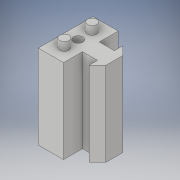
# Autodesk Inventor part: Grab Rail v2
Saved by Autodesk Inventor 2018 (Build 220112000, 112)
## iProperties
Created: 2019-12-11
Part Number: Grab Rail v2
Material: Generic
Document SubType Name: Modeling
Designer: AOFUser
Density: 1 g/cm^3
Appearance: Default
Author: AOFUser
Autodesk Inventor part; units mm, degrees
ref_plane "YZ Plane" through (0, 0, 0) normal (1, 0, 0) x (0, 1, 0)
ref_plane "XZ Plane" through (0, 0, 0) normal (0, 1, 0) x (-1, 0, 0)
ref_plane "XY Plane" through (0, 0, 0) normal (0, 0, 1) x (1, 0, 0)
sketch "Sketch1" plane through (0, 0, 0) normal (0, 1, 0) x (-1, 0, 0)
  line L0 (0, 0) -> (7.62, 0)
  line L1 (7.62, 0) -> (7.62, -16.51)
  line L2 (7.62, -16.51) -> (0, -16.51)
  line L3 (0, -16.51) -> (0, 0)
  line L4 (0, 0) -> (0, -5.715)
  line L5 (0, -5.715) -> (-7.112, -5.715)
  line L6 (-7.112, -5.715) -> (-7.112, -10.795)
  line L7 (-7.112, -10.795) -> (0, -10.795)
  line L8 (-7.112, -5.715) -> (-4.572, -5.715)
  line L9 (-4.572, -5.715) -> (-4.572, -3.175)
  line L10 (-4.572, -3.175) -> (-7.112, -5.715)
  line L11 (-7.112, -10.795) -> (-4.572, -10.795)
  line L12 (-4.572, -10.795) -> (-4.572, -13.335)
  line L13 (-4.572, -13.335) -> (-7.112, -10.795)
  dimension "d0" = 7.62
  dimension "d1" = 16.51
  dimension "d2" = 5.715
  dimension "d3" = 7.112
  dimension "d4" = 5.08
  dimension "d5" = 2.54
  dimension "d6" = 2.54
  dimension "d7" = 2.54
  constraints: 28 end point, 5 perpendicular, 5 point on line, 2 horizontal, 2 parallel
  measures "d0" distance of L1.end L2.end
  measures "d1" distance of L0.end L1.end
  measures "d2" distance of L0.start L4.end
  measures "d3" distance of L4.end L5.end
  measures "d4" distance of L5.end L6.end
  measures "d5" distance of L5.end L8.end
  measures "d6" distance of L8.end L9.end
  measures "d7" distance of L11.end L12.end
extrude "Extrusion1" add sketch "Sketch1" along normal blind 25.4
sketch "Sketch2" plane through (0, 25.4, 0) normal (0, 1, 0) x (1, 0, 0)
  line L0 (-7.62, 0) -> (0, 0) projected
  line L1 (-3.81, 0) -> (-3.81, 4.064)
  line L2 (0, 16.51) -> (-7.62, 16.51) projected
  line L3 (-3.81, 16.51) -> (-3.81, 12.446)
  circle A0 centre (-3.81, 4.064) radius 1.397
  circle A1 centre (-3.81, 12.446) radius 1.397
  dimension "d10" = 4.064
  dimension "d11" = 4.064
  dimension "d12" = 2.794
  dimension "d13" = 2.794
  constraints: 4 end point, 2 centre point, 2 coincident, 2 midpoint, 2 vertical
  measures "d10" distance of L1.start L1.end
  measures "d11" distance of L3.start L3.end
  measures "d12" diameter of A0
  measures "d13" diameter of A1
extrude "Extrusion2" add sketch "Sketch2" along normal blind 2.54
sketch "Sketch3" plane through (0, 25.4, 0) normal (0, 1, 0) x (1, 0, 0)
  line L0 (-7.62, 0) -> (0, 0) projected
  line L1 (-3.81, 0) -> (-3.81, 8.255)
  dimension "d16" = 8.255
  constraints: 2 end point, 1 midpoint, 1 vertical
  measures "d16" distance of L1.start L1.end
hole "Hole1" at (-3.81, 25.4, -8.255) direction (0, -1, 0) diameter 2.794 depth 11.43 tip angle 118
body "Solid1"
